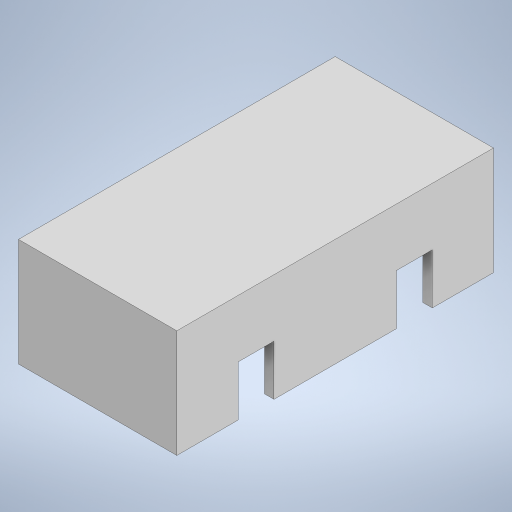
# Autodesk Inventor part: Suporte Eletroimã
Saved by Autodesk Inventor 2023 (Build 270158000, 158)
## iProperties
Created: 2023-03-07
Part Number: Suporte Eletroimã
Material: Genérico
Document SubType Name: Modeling
Designer: Inteli
Density: 1 g/cm^3
Appearance: Padrão
Author: Inteli
Autodesk Inventor part; units mm, degrees
ref_plane "YZ Plane" through (0, 0, 0) normal (1, 0, 0) x (0, 1, 0)
ref_plane "XZ Plane" through (0, 0, 0) normal (0, 1, 0) x (-1, 0, 0)
ref_plane "XY Plane" through (0, 0, 0) normal (0, 0, 1) x (1, 0, 0)
sketch "Esboço1" plane through (0, 0, 0) normal (0, 1, 0) x (-1, 0, 0)
  circle A0 centre (0, 11) radius 10
  circle A1 centre (0, -11) radius 10
  line L0 (9, 2) -> (-9, 2)
  line L1 (-9, -2) -> (9, -2)
  line L2 (9, 20) -> (-9, 20)
  line L3 (-9, -20) -> (9, -20)
  line L4 (11, 22) -> (-11, 22)
  line L5 (-11, 22) -> (-11, -22)
  line L6 (-11, -22) -> (11, -22)
  line L7 (11, -22) -> (11, 22)
  line L8 (9, -20) -> (9, -2)
  line L9 (9, 2) -> (9, 20)
  line L10 (-9, 20) -> (-9, 2)
  line L11 (-9, -2) -> (-9, -20)
  point P0 (0, 0)
  point P1 (0, 0)
  point P2 (-9, 6.6411)
  point P3 (-9, 15.3589)
  point P4 (-4.3589, 20)
  point P5 (4.3589, 20)
  point P6 (9, 15.3589)
  point P7 (9, 6.6411)
  point P8 (4.3589, 2)
  point P9 (-4.3589, 2)
  point P10 (-9, -6.6411)
  point P11 (-4.3589, -2)
  point P12 (4.3589, -2)
  point P13 (9, -6.6411)
  point P14 (9, -15.3589)
  point P15 (4.3589, -20)
  point P16 (-4.3589, -20)
  point P17 (-9, -15.3589)
  dimension "d15" = 22
  dimension "d16" = 40
  dimension "d17" = 18
  dimension "d18" = 22
  dimension "d19" = 44
  constraints: 24 end point, 8 parallel, 3 horizontal, 3 perpendicular, 2 centre point, 1 coincident
  measures "d15" distance of A1.centre point (0, 11)
  measures "d16" distance of L3.start L2.end
  measures "d17" distance of L3.start L3.end
  measures "d18" distance of L6.end L5.end
  measures "d19" distance of L5.end L4.end
extrude "Base Principal dos Imãs" add sketch "Esboço1" along normal blind 13
sketch "Esboço2" plane through (11, 0, 22) normal (1, 0, 0) x (0, 0, -1)
  line L0 (13.5, 7) -> (13.5, 0)
  line L1 (8.5, 7) -> (8.5, 0)
  line L2 (30.5, 7) -> (30.5, 0)
  line L3 (35.5, 7) -> (35.5, 0)
  line L4 (8.5, 7) -> (13.5, 7)
  line L5 (30.5, 7) -> (35.5, 7)
  line L6 (8.5, 0) -> (13.5, 0)
  line L7 (6.6411, 0) -> (15.3589, 0) projected
  line L8 (30.5, 0) -> (35.5, 0)
  point P0 (22, 0)
  constraints: 16 end point, 2 perpendicular, 2 point on line, 1 collinear
extrude "Rasgo Fios Imãs" cut sketch "Esboço2" against normal up to surface (2 mm away)
sketch "Esboço3" plane through (0, 13, 0) normal (0, 1, 0) x (1, 0, 0)
  line L0 (11, -22) -> (11, 22) projected
  line L1 (-11, -22) -> (11, -22)
  line L2 (11, -22) -> (11, 22)
  line L3 (11, 22) -> (-11, 22)
  line L4 (-11, 22) -> (-11, -22)
  line L5 (-11, -22) -> (11, 22) construction
  line L6 (11, -22) -> (-11, 22) construction
  point P0 (0, 0)
  constraints: 12 end point, 2 midpoint, 2 parallel, 1 horizontal, 1 perpendicular
extrude "Extrusão3" add sketch "Esboço3" along normal blind 2
